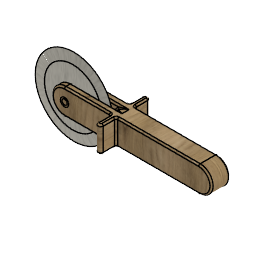
Pizza Cutter (Autodesk Fusion 360 design; units mm, degrees)
part number: 2026-06-11-20-28-39-290
Autodesk Fusion 360 part; units mm, degrees
note: some values were not read from the file. Set by a fixed rule: which face or edge a step refers to.
sketch "Sketch1" plane through (0, 0, 0) normal (0, 1, 0) x (1, 0, 0)
  line L0 (50, -12.5) -> (130, -12.5)
  arc A0 (130, -12.5) -> (130, 12.5) centre (130, 0) ccw
  line L1 (130, 12.5) -> (50, 12.5)
  arc A1 (50, 12.5) -> (50, -12.5) centre (50, 0) ccw
  line L2 (50, 0) -> (130, 0) construction
  dimension "d1" = 80
  dimension "d2" = 12.5
  dimension "d3" = 50
  constraint tangent L0 A0
  constraint tangent A0 L1
  constraint parallel L0 L1
  constraint tangent L1 A1
  constraint tangent L0 A1
  constraint horizontal L2
  constraint coincident origin L2
  measures "d1" distance of L0.start L0.end
  measures "d2" radius of A0
  measures "d3" horizontal distance of origin A1.centre
extrude "Extrude1" add sketch "Sketch1" against normal blind 2 makes body 1
sketch "Sketch2" plane through (0, -2, 0) normal (0, -1, 0) x (1, 0, 0)
  arc A0 (50, 12.5) -> (50, -12.5) centre (50, 0) ccw
  line L0 (50, -12.5) -> (130, -12.5)
  arc A1 (130, -12.5) -> (130, 12.5) centre (130, 0) ccw
  line L1 (130, 12.5) -> (50, 12.5)
  line L2 (130, 12.5) -> (0, 12.5)
  arc A2 (0, 12.5) -> (0, -12.5) centre (0, 0) ccw
  line L3 (0, -12.5) -> (130, -12.5)
  arc A3 (130, -12.5) -> (130, 12.5) centre (130, 0) ccw
  line L4 (130, 0) -> (0, 0) construction
  circle A4 centre (0, 0) radius 2.5
  dimension "d6" = 25
  dimension "d7" = 5
  constraint tangent L2 A2
  constraint tangent A2 L3
  constraint parallel L2 L3
  constraint tangent L3 A3
  constraint tangent L2 A3
  constraint coincident A2.centre L4.end
  constraint horizontal L4
  constraint coincident A1.centre A3.centre
  constraint concentric A2 A4
  measures "d6" diameter of A2
  measures "d7" diameter of A4
extrude "Extrude2" add sketch "Sketch2" along normal blind 7 bodies 1
sketch "Sketch3" plane through (0, -9, 0) normal (0, -1, 0) x (1, 0, 0)
  circle A0 centre (0, 0) radius 2.5
  arc A1 (130, -12.5) -> (130, 12.5) centre (130, 0) ccw
  line L0 (130, 12.5) -> (0, 12.5)
  arc A2 (0, 12.5) -> (0, -12.5) centre (0, 0) ccw
  line L1 (0, -12.5) -> (130, -12.5)
  line L2 (45, 12.5) -> (50, 12.5)
  line L3 (50, 12.5) -> (50, -12.5)
  line L4 (50, -12.5) -> (45, -12.5)
  line L5 (45, -12.5) -> (45, 12.5)
  dimension "d10" = 5
  dimension "d11" = 45
  constraint horizontal L2
  constraint vertical L3
  constraint horizontal L4
  constraint vertical L5
  constraint coincident L1 L3.end
  constraint coincident L0 L2.start
  measures "d10" distance of L2.start L2.end
  measures "d11" horizontal distance of L2.start A0.centre
extrude "Extrude3" add sketch "Sketch3" along normal blind 15 contours L0 L1 L2 L3 L4 L5 bodies 1
fillet "Fillet1" radius 2.5 2 edges at (50, -24, 0) (45, -24, 0) on bodies 1
mirror "Mirror1" about plane through (0, 0, 0) normal (0, 1, 0) of bodies 1 merged
fillet "Fillet2" radius 1.5 40 edges at (50, -9, 0) (50, -15.25, 12.5) (47.5, -24, 12.5) (45, -15.25, 12.5) (45, 15.25, -12.5) (47.5, 24, -12.5) (50, 15.25, -12.5) (50, 9, 0) (-2.3308, -2, 0.904) (22.5, 9, 12.5) (-12.5, 9, 0) (22.5, 9, -12.5) (90, -9, -12.5) (142.5, -9, 0) (90, -9, 12.5) (50, -15.25, -12.5) (47.5, -24, -12.5) (45, -15.25, -12.5) (37.5, -2, 0) (-2.3308, -9, 0.904) (45, -9, 0) (45, 9, 0) (-2.3308, 9, 0.904) (50, 15.25, 12.5) (47.5, 24, 12.5) (45, 15.25, 12.5) (22.5, -9, 12.5) (-12.5, -9, 0) (22.5, -9, -12.5) (-2.3308, 2, 0.904) (25, 2, 12.5) (-12.5, 2, 0) (25, 2, -12.5) (90, 9, -12.5) (142.5, 9, 0) (90, 9, 12.5) (37.5, 2, 0) (25, -2, 12.5) (-12.5, -2, 0) (25, -2, -12.5) 20 faces at (45.5348, -23.0456, -4.1667) (45, -13.1668, -4.1667) (50, -13.1668, 4.1667) (103.3333, -9, -4.1667) (30.8333, -9, 0) (2.4876, -6.6667, -0.2489) (45.5348, 23.0456, -4.1667) (50, 13.1668, 4.1667) (45, 13.1668, -4.1667) (2.4876, 6.6667, -0.2489) (103.3333, 9, -4.1667) (13.5388, -2, 6.0505) (13.5388, 2, 6.0505) (103.3333, 0.6667, -12.5) (-9.3723, -4.3333, -8.2711) (103.3333, -0.6667, 12.5) (136.5179, -3, -10.6661) (-9.3723, 4.3333, -8.2711) (43.4821, -0.6667, 10.6661) (30.8333, 9, 0) on bodies 1
sketch "Sketch4" plane through (0, 0, 0) normal (0, 1, 0) x (1, 0, 0)
  circle A0 centre (0, 0) radius 2.5
  dimension "d20" = 5
  constraint coincident A0.centre origin
  measures "d20" diameter of A0
extrude "Extrude4" add sketch "Sketch4" along normal mid plane 18 separate body makes body 2
sketch "Sketch5" plane through (0, 0, 0) normal (1, 0, 0) x (0, 1, 0)
  line L0 (0, 2.5) -> (-1, 2.5)
  line L1 (-1, 2.5) -> (-1, 27.5)
  line L2 (-1, 27.5) -> (0, 37.5)
  line L3 (0, 37.5) -> (0, 2.5)
  line L4 (1, 2.5) -> (1, 27.5)
  line L5 (1, 27.5) -> (0, 37.5)
  line L6 (0, 2.5) -> (1, 2.5)
  line L7 (0, 37.5) -> (0, 2.5)
  dimension "d23" = 35
  dimension "d24" = 10
  dimension "d25" = 2.5
  dimension "d26" = 1
  constraint horizontal L0
  constraint perpendicular L0 L1
  constraint perpendicular L0 L3
  constraint coincident origin L3
  constraint symmetric L0.start L3 L6.start
  constraint symmetric L0.end L3 L4.start
  constraint symmetric L1.end L3 L4.end
  constraint symmetric L2.end L3 L5.end
  measures "d23" distance of L0.start L2.end
  measures "d24" vertical distance of L1.end L2.end
  measures "d25" distance of origin L0.start
  measures "d26" distance of L1 L3
revolve "Revolve1" add sketch "Sketch5" angle 360 about axis through (0, 1.75, 0) along (0, 1, 0) bodies 1 2
